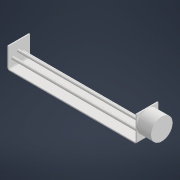
# Autodesk Inventor part: 026
Saved by Autodesk Inventor 2022 (Build 260153000, 153)
## iProperties
Created: 2022-04-02
Part Number: 026
Material: Stainless Steel, 440C
Document SubType Name: Sheet Metal
Designer: Vinicius Miguel
Density: 7.75 g/cm^3
Sheet Metal Rule: Default_mm
Appearance: Semi-Polished
Author: Vinicius Miguel
Autodesk Inventor part; units mm, degrees
ref_plane "YZ Plane" through (0, 0, 0) normal (1, 0, 0) x (0, 1, 0)
ref_plane "XZ Plane" through (0, 0, 0) normal (0, 1, 0) x (-1, 0, 0)
ref_plane "XY Plane" through (0, 0, 0) normal (0, 0, 1) x (1, 0, 0)
sketch "Sketch1" plane through (0, 0, 0) normal (0, 1, 0) x (-1, 0, 0)
  line L0 (45, 7.5) -> (-45, 7.5)
  line L1 (-45, 7.5) -> (-45, -7.5)
  line L2 (-45, -7.5) -> (45, -7.5)
  line L3 (45, -7.5) -> (45, 7.5)
  line L4 (45, 7.5) -> (-45, -7.5) construction
  line L5 (-45, 7.5) -> (45, -7.5) construction
  point P0 (0, 0)
  dimension "d0" = 90
  dimension "d1" = 15
  measures "d0" distance of L2.end L1.end
  measures "d1" distance of L1.end L0.end
extrude "Plate1" add sketch "Sketch1" along normal blind 0.75
sketch "Sketch2" plane through (-44.25, 0, 7.5) normal (-1, 0, 0) x (0, -1, 0)
  line L0 (0, -15) -> (0, 0)
  line L1 (0, 0) -> (-14.5, 0)
  line L2 (-14.5, 0) -> (-14.5, -15)
  line L3 (-14.5, -15) -> (0, -15)
  constraints: 6 end point, 1 horizontal, 1 perpendicular, 1 vertical
edge flange "Flange1" height 14.5 angle 90 thickness 0.75 bend radius 0.75 thickness toward (-1, 0, 0) relief tear relief width 0.75 relief depth 0.375 edges at (-45, 0.75, 0) wall of the first edge with corners at (-44.25, 0, -7.5) (-44.25, 0, 7.5) (-44.25, 14.5, 7.5) (-44.25, 14.5, -7.5)
bend "Bend1"
corner "Corner1"
sketch "Sketch3" plane through (44.25, 0, -7.5) normal (1, 0, 0) x (0, 1, 0)
  line L0 (0, 15) -> (0, 0)
  line L1 (0, 0) -> (18, 0)
  line L2 (18, 0) -> (18, 15)
  line L3 (18, 15) -> (0, 15)
  constraints: 6 end point, 1 horizontal, 1 perpendicular, 1 vertical
edge flange "Flange2" height 18 angle 90 thickness 0.75 bend radius 0.75 thickness toward (1, 0, 0) relief tear relief width 0.75 relief depth 0.375 edges at (45, 0.75, 0) wall of the first edge with corners at (44.25, 0, 7.5) (44.25, 0, -7.5) (44.25, 18, -7.5) (44.25, 18, 7.5)
bend "Bend2"
corner "Corner2"
sketch "Sketch4" plane through (45, 18, 7.5) normal (1, 0, 0) x (0, 0, -1)
  circle A0 centre (7.5, -7.5) radius 7.5
  point P0 (7.5, -18)
  dimension "d23" = 10.5
  dimension "d24" = 15
  constraints: 1 centre point, 1 coincident, 1 vertical alignment
  measures "d23" distance of point (7.5, -18) point (7.5, -7.5)
  measures "d24" diameter of A0
extrude "Extrusion1" add sketch "Sketch4" along normal blind 10
sketch "Sketch5" plane through (-45, 14.5, -7.5) normal (-1, 0, 0) x (0, 0, 1)
  circle A0 centre (7.5, -4) radius 1.5
  circle A1 centre (12.5, -8) radius 1.5
  circle A2 centre (2.5, -8) radius 1.5
  point P0 (7.5, -14.5)
  dimension "d29" = 10.5
  dimension "d30" = 3
  dimension "d31" = 3
  dimension "d32" = 3
  dimension "d33" = 5
  dimension "d34" = 5
  dimension "d35" = 4
  constraints: 3 centre point, 1 horizontal alignment, 1 vertical alignment
  measures "d29" distance of A0.centre point (7.5, -14.5)
  measures "d30" diameter of A0
  measures "d31" diameter of A1
  measures "d32" diameter of A2
  measures "d33" horizontal distance of A0.centre A2.centre
  measures "d34" horizontal distance of A0.centre A1.centre
  measures "d35" vertical distance of A0.centre A1.centre
extrude "Extrusion2" add sketch "Sketch5" against normal up to surface (89.25 mm away)
equation "\"d34\" = d33"
equation "\"d2\" = Thickness"
equation "\"d3\" = BendReliefWidth"
equation "\"d4\" = BendReliefDepth"
equation "\"d5\" = MinimumRemnant"
equation "\"d6\" = TransitionRadius"
equation "\"d9\" = BendRadius"
equation "\"d10\" = CornerReliefSize"
equation "\"d11\" = GapSize"
equation "\"d12\" = JacobiRadiusSize"
equation "\"d13\" = BendReliefWidth"
equation "\"d14\" = BendReliefDepth"
equation "\"d15\" = MinimumRemnant"
equation "\"d16\" = TransitionRadius"
equation "\"d19\" = BendRadius"
equation "\"d20\" = CornerReliefSize"
equation "\"d21\" = GapSize"
equation "\"d22\" = JacobiRadiusSize"
equation "\"BendRadius\" = Thickness"
equation "\"BendReliefWidth\" = Thickness"
equation "\"BendReliefDepth\" = 0.5 * Thickness"
equation "\"CornerReliefSize\" = 4 * Thickness"
equation "\"MinimumRemnant\" = 2 * Thickness"
equation "\"TransitionRadius\" = BendRadius"
equation "\"JacobiRadiusSize\" = BendRadius"
equation "\"GapSize\" = Thickness"
equation "\"Thickness\" = 0.75"
body "Solid1"
